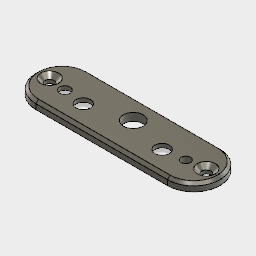
NuTube Skittle Ver.2 (Autodesk Fusion 360 design; units mm, degrees)
Autodesk Fusion 360 part; units mm, degrees
note: some values were not read from the file. Set by a fixed rule: the direction of a hole.
sketch "スケッチ1" plane through (0, 0, 0) normal (0, 1, 0) x (1, 0, 0)
  line L0 (-25, -10) -> (25, -10)
  arc A0 (25, -10) -> (25, 10) centre (25, 0) ccw
  line L1 (25, 10) -> (-25, 10)
  arc A1 (-25, 10) -> (-25, -10) centre (-25, 0) ccw
  line L2 (-25, 0) -> (25, 0) construction
  line L3 (-23, 10) -> (-23, -10) construction
  line L4 (-15, 10) -> (-15, -10) construction
  line L5 (15, 10) -> (15, -10) construction
  line L6 (23, 10) -> (23, -10) construction
  line L7 (-23, -1) -> (23, -1) construction
  line L8 (-15, -2) -> (15, -2) construction
  line L9 (0, 10) -> (0, -10) construction
  line L10 (-24.25, -0.25) -> (-24.25, -1.75)
  arc A2 (-24.25, -1.75) -> (-21.75, -1.75) centre (-23, -1.75) ccw
  line L11 (-21.75, -1.75) -> (-21.75, -0.25)
  arc A3 (-21.75, -0.25) -> (-24.25, -0.25) centre (-23, -0.25) ccw
  line L12 (-23, -0.25) -> (-23, -1.75) construction
  point P0 (-35, 0)
  point P1 (35, 0)
  point P2 (-23, -1)
  point P3 (-15, -2)
  point P4 (15, -2)
  point P5 (23, -1)
  point P6 (0, 2)
  point P7 (0, -4)
  point P8 (-23, -1)
  point P9 (-23, 1)
  point P10 (-23, -3)
  dimension "d1" = 20
  dimension "d2" = 70
  dimension "d13" = 6
  dimension "d14" = 12
  dimension "d15" = 9
  dimension "d16" = 8
  dimension "d17" = 15
  dimension "d18" = 15
  dimension "d19" = 23
  dimension "d20" = 23
  dimension "d40" = 4
  dimension "d41" = 2.5
  measures "d1" distance of L0 L1
  measures "d2" distance of P0 P1
  measures "d13" distance of L0 P7
  measures "d14" distance of L0 P6
  measures "d15" distance of L0 L7
  measures "d16" distance of L0 L8
  measures "d17" distance of L4 L9
  measures "d18" distance of L5 L9
  measures "d19" distance of L3 L9
  measures "d20" distance of L6 L9
  measures "d40" distance of P9 P10
  measures "d41" distance of L10 L11
extrude "押し出し1" add sketch "スケッチ1" along normal blind 3 contours L0 A0 L1 A1 | L10 A2 L11 A3
chamfer "面取り1" distance 1 angle 45 4 edges at (0, 3, -10) (-35, 3, 0) (0, 3, 10) (35, 3, 0)
sketch "スケッチ2" plane through (0, 3, 0) normal (0, 1, 0) x (-1, 0, 0)
  line L0 (-25, -9) -> (25, -9)
  arc A0 (25, -9) -> (25, 9) centre (25, 0) ccw
  line L1 (25, 9) -> (-25, 9)
  arc A1 (-25, 9) -> (-25, -9) centre (-25, 0) ccw
  arc A2 (25, -10) -> (25, 10) centre (25, 0) ccw
  line L2 (-25, -10) -> (25, -10)
  arc A3 (-25, 10) -> (-25, -10) centre (-25, 0) ccw
  line L3 (25, 10) -> (-25, 10)
  line L4 (35, 0) -> (-35, 0) construction
  point P0 (29.8, 0)
  point P1 (-29.8, 0)
  dimension "d6" = 5.2
  dimension "d7" = 5.2
  measures "d6" distance of L4.start P0
  measures "d7" distance of L4.end P1
hole "穴1" at (-29.8, 3, 0) at (29.8, 3, 0) direction (0, -1, 0) diameter 3.5 end through all countersink diameter 6.8 countersink angle 90
hole "穴2" at (0, 0, -2) direction (0, 1, 0) diameter 7.5 end through all
hole "穴3" at (0, 0, 4) direction (0, 1, 0) diameter 2 depth 1 tip angle 180
hole "穴4" at (-15, 0, 2) at (15, 0, 2) direction (0, 1, 0) diameter 5.5 end through all counterbore diameter 10 counterbore depth 1.5
hole "穴5" at (-23, 0, 1) direction (0, 1, 0) diameter 4 end through all counterbore diameter 9 counterbore depth 1.5
hole "穴6" at (23, 0, 1) direction (0, 1, 0) diameter 3.5 end through all
